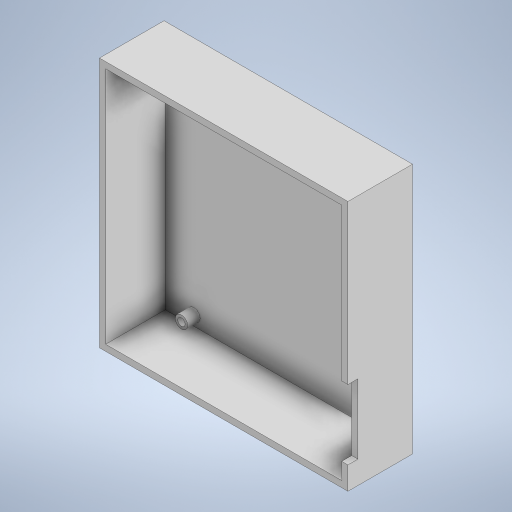
# Autodesk Inventor part: Base ESP
Saved by Autodesk Inventor 2023 (Build 270158000, 158)
## iProperties
Created: 2022-12-12
Part Number: Base ESP
Material: Genérico
Document SubType Name: Modeling
Designer: Inteli
Density: 1 g/cm^3
Appearance: Padrão
Author: Inteli
## iProperties of the stored document Base ESP_3DPrint.ipt
Created: 2022-12-13
Part Number: Base ESP_3DPrint
Material: Genérico
Document SubType Name: Modeling
Designer: Inteli
Density: 1 g/cm^3
Appearance: Padrão
Author: Inteli
Autodesk Inventor part; units mm, degrees
ref_plane "YZ Plane" through (0, 0, 0) normal (1, 0, 0) x (0, 1, 0)
ref_plane "XZ Plane" through (0, 0, 0) normal (0, 1, 0) x (-1, 0, 0)
ref_plane "XY Plane" through (0, 0, 0) normal (0, 0, 1) x (1, 0, 0)
sketch "Esboço1" plane through (0, 0, 0) normal (0, 0, 1) x (1, 0, 0)
  line L0 (-50, 50.5) -> (50, 50.5)
  line L1 (50, 50.5) -> (50, -50.5)
  line L2 (50, -50.5) -> (-50, -50.5)
  line L3 (-50, -50.5) -> (-50, 50.5)
  line L4 (-50, 50.5) -> (50, -50.5) construction
  line L5 (50, 50.5) -> (-50, -50.5) construction
  point P0 (0, 0)
  dimension "d0" = 100
  dimension "d1" = 101
  constraints: 12 end point, 2 midpoint, 2 parallel, 1 horizontal, 1 perpendicular
  measures "d0" distance of L1.end L2.end
  measures "d1" distance of L0.end L1.end
extrude "Base" add sketch "Esboço1" along normal blind 26
sketch "Esboço2" plane through (0, 0, 26) normal (0, 0, 1) x (1, 0, 0)
  line L0 (50, 50.5) -> (-50, 50.5) projected
  line L1 (-50, -50.5) -> (50, -50.5) projected
  line L2 (-50, 50.5) -> (50, 50.5)
  line L3 (50, 50.5) -> (50, -50.5)
  line L4 (50, -50.5) -> (-50, -50.5)
  line L5 (-50, -50.5) -> (-50, 50.5)
  line L6 (47.5, -48) -> (47.5, 48)
  line L7 (47.5, 48) -> (-47.5, 48)
  line L8 (-47.5, 48) -> (-47.5, -48)
  line L9 (-47.5, -48) -> (47.5, -48)
  point P0 (0, 0)
  dimension "d4" = 2.5
  constraints: 16 end point, 4 parallel, 2 perpendicular, 1 horizontal, 3 other
  measures "d4" distance between parallel lines of L3 L6
extrude "Área" cut sketch "Esboço2" against normal blind 24 contours L9 L8 L7 L6
sketch "Esboço3" plane through (0, 0, 2) normal (0, 0, 1) x (1, 0, 0)
  circle A0 centre (-36, -44) radius 1.5
  line L0 (-50, 50.5) -> (-50, -50.5) projected
  line L1 (-50, -50.5) -> (50, -50.5) projected
  line L2 (-47.5, -48) -> (-47.5, 48) projected
  line L3 (47.5, 48) -> (47.5, -48) projected
  circle A1 centre (-36, 44) radius 1.5
  circle A2 centre (36, -44) radius 1.5
  circle A3 centre (36, 44) radius 1.5
  circle A4 centre (-36, -44) radius 2.5
  line L4 (47.5, -48) -> (-47.5, -48) projected
  line L5 (-47.5, 48) -> (47.5, 48) projected
  circle A5 centre (-36, 44) radius 2.5
  circle A6 centre (36, -44) radius 2.5
  circle A7 centre (36, 44) radius 2.5
  dimension "d11" = 3
  dimension "d12" = 14
  dimension "d13" = 6.5
  dimension "d14" = 5
  constraints: 8 centre point, 3 coincident
  measures "d11" diameter of A0
  measures "d12" distance from line of L0 A0.centre
  measures "d13" distance from line of L1 A0.centre
  measures "d14" diameter of A4
extrude "Extrusão3" add sketch "Esboço3" along normal blind 5 contours A4 | A5 | A6 | A7
sketch "Esboço4" plane through (50, -50.5, 0) normal (1, 0, 0) x (0, 0, -1)
  line L0 (-26, 9.2) -> (-22, 9.2)
  line L1 (-22, 9.2) -> (-22, 37.2)
  line L2 (-22, 37.2) -> (-26, 37.2)
  line L3 (-26, 37.2) -> (-26, 9.2)
  point P0 (0, 50.5)
  dimension "d17" = 4
  dimension "d18" = 28
  constraints: 8 end point, 2 parallel, 1 horizontal, 1 perpendicular
  measures "d17" distance of L2.end L1.end
  measures "d18" distance of L1.end L0.end
extrude "Extrusão4" cut sketch "Esboço4" against normal up to surface (2.5 mm away)
